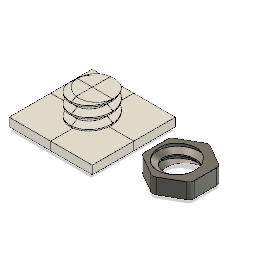
TileLinkTest1 (Autodesk Fusion 360 design; units mm, degrees)
Autodesk Fusion 360 part; units mm, degrees
sketch "Sketch1" plane through (0, 0, 0) normal (0, 1, 0) x (1, 0, 0)
  line L0 (40, 40) -> (-40, 40)
  line L1 (-40, 40) -> (-40, -40)
  line L2 (-40, -40) -> (40, -40)
  line L3 (40, -40) -> (40, 40)
  line L4 (40, 40) -> (-40, -40) construction
  line L5 (-40, 40) -> (40, -40) construction
  dimension "d1" = 80
  dimension "d2" = 80
extrude "Extrude1" add sketch "Sketch1" along normal blind 8.196 makes body 1
sketch "Sketch2" plane through (0, 8.196, 0) normal (0, 1, 0) x (-1, 0, 0)
  line L0 (-40, 40) -> (-40, -40)
  line L1 (-40, -40) -> (40, -40)
  line L2 (40, -40) -> (40, 40)
  line L3 (40, 40) -> (-40, 40)
  circle A0 centre (0, 0) radius 20
  dimension "d5" = 40
  measures "d5" diameter of A0
extrude "Extrude2" add sketch "Sketch2" along normal blind 25 contours A0 bodies 1
thread "Thread1" "ISO Metric Trapezoidal Threads 40.0 TR40x10 7e" major diameter 39.735 minor diameter 28.675 pitch 10 angle 60 modelled right hand crest width 1.25 on face at (-19.9006, 16.5293, -1.9914) crest through (-19.8675, 7.571, 0) on bodies 1
ref_plane "WorkPlane1" through (0, 4.098, 0) normal (0, 0, 1) x (1, 0, 0)
split "Split1" by plane through (0, 4.098, 0) normal (0, 0, 1) bodies 1 makes body 2 at (13.3333, 0, 26.6667)
ref_plane "WorkPlane2" through (0, 4.098, 20) normal (-1, 0, 0) x (0, 0, 1)
split "Split2" by plane through (0, 4.098, 20) normal (-1, 0, 0) bodies 1 2 makes body 4 at (-26.6667, 0, 13.3333) makes body 3 at (-26.6667, 0, -26.6667)
sketch "Sketch3" plane through (0, 0, 0) normal (0, 1, 0) x (1, 0, 0)
  circle A0 centre (85, 0) radius 27.5
  circle A1 centre (85, 0) radius 18.0278
  line L0 (85, 27.5) -> (61.1843, 13.75)
  line L1 (61.1843, 13.75) -> (61.1843, -13.75)
  line L2 (61.1843, -13.75) -> (85, -27.5)
  line L3 (85, -27.5) -> (108.8157, -13.75)
  line L4 (108.8157, -13.75) -> (108.8157, 13.75)
  line L5 (108.8157, 13.75) -> (85, 27.5)
  dimension "d8" = 55
  measures "d8" diameter of A0
extrude "Extrude3" add sketch "Sketch3" along normal blind 15 separate body contours L0 L1 L2 L3 L4 L5 makes body 5
thread "Thread2" "ISO Metric Trapezoidal Threads 40.0 TR40x10 7H" major diameter 41 minor diameter 30.355 pitch 10 angle 60 modelled right hand crest width 1.25 on face at (103.0053, 5, 0.8986) crest through (100.1775, -5.625, 0) on bodies 5
fillet "Fillet1" radius 5 6 edges at (61.1843, 7.5, 13.75) (85, 7.5, 27.5) (108.8157, 7.5, 13.75) (108.8157, 7.5, -13.75) (61.1843, 7.5, -13.75) (85, 7.5, -27.5) on bodies 5
